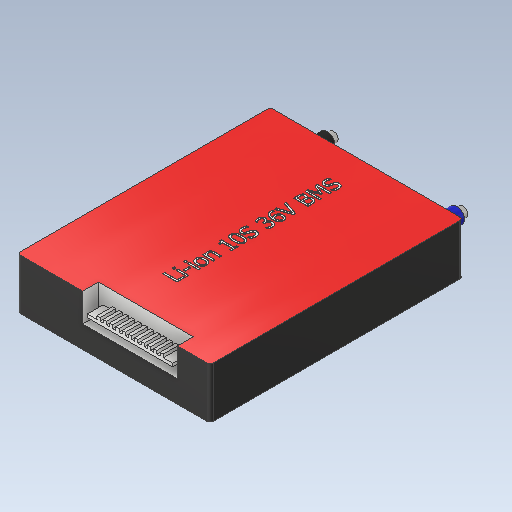
# Autodesk Inventor part: BMS
Saved by Autodesk Inventor 2020.1 (Build 241239000, 239)
## iProperties
Created: 2019-07-12
Part Number: BMS
Material: Generic
Document SubType Name: Modeling
Designer: Petar
Density: 1 g/cm^3
Appearance: Default
Author: Petar
Autodesk Inventor part; units mm, degrees
ref_plane "YZ Plane" through (0, 0, 0) normal (1, 0, 0) x (0, 1, 0)
ref_plane "XZ Plane" through (0, 0, 0) normal (0, 1, 0) x (-1, 0, 0)
ref_plane "XY Plane" through (0, 0, 0) normal (0, 0, 1) x (1, 0, 0)
sketch "Sketch1" plane through (0, 0, 0) normal (0, 1, 0) x (-1, 0, 0)
  line L0 (-30.5, 40) -> (30.5, 40)
  line L1 (30.5, 40) -> (30.5, -40)
  line L2 (30.5, -40) -> (-30.5, -40)
  line L3 (-30.5, -40) -> (-30.5, 40)
  line L4 (-30.5, 40) -> (30.5, -40) construction
  line L5 (30.5, 40) -> (-30.5, -40) construction
  point P0 (0, 0)
  dimension "d0" = 61
  dimension "d1" = 80
  constraints: 12 end point, 2 midpoint, 2 parallel, 1 horizontal, 1 perpendicular
  measures "d0" distance of L1.end L2.end
  measures "d1" distance of L0.end L1.end
extrude "Extrusion1" add sketch "Sketch1" along normal blind 16
sketch "Sketch2" plane through (0, 16, 0) normal (0, 1, 0) x (1, 0, 0)
  line L0 (-3.4837, -32.5737) -> (-3.4837, 39.7617) construction
  line L1 (-3.4837, 39.7617) -> (4.1906, 39.7617) construction
  line L2 (4.1906, 39.7617) -> (4.1906, -32.5737) construction
  line L3 (4.1906, -32.5737) -> (-3.4837, -32.5737) construction
  line L4 (-30.5, -40) -> (30.5, -40) construction
  line L5 (-9.8385, -40) -> (20.1615, -40)
  line L6 (20.1615, -40) -> (20.1615, -35)
  line L7 (20.1615, -35) -> (-9.8385, -35)
  line L8 (-9.8385, -35) -> (-9.8385, -40)
  line L9 (2.6034, -19.9781) -> (2.6034, -22.5855)
  line L10 (2.6034, -22.5855) -> (-1.8966, -22.5855)
  line L11 (-1.8966, -22.5855) -> (-1.8966, -21.9874)
  line L12 (-1.8966, -21.9874) -> (2.071, -21.9874)
  line L13 (2.071, -21.9874) -> (2.071, -19.9781)
  line L14 (2.071, -19.9781) -> (2.6034, -19.9781)
  line L15 (2.6034, -18.9716) -> (2.6034, -19.5405)
  line L16 (2.6034, -19.5405) -> (-0.7734, -19.5405)
  line L17 (-0.7734, -19.5405) -> (-0.7734, -18.9716)
  line L18 (-0.7734, -18.9716) -> (2.6034, -18.9716)
  line L19 (-1.335, -18.9315) -> (-1.335, -19.577)
  line L20 (-1.335, -19.577) -> (-1.9257, -19.577)
  line L21 (-1.9257, -19.577) -> (-1.9257, -18.9315)
  line L22 (-1.9257, -18.9315) -> (-1.335, -18.9315)
  line L23 (0.9077, -16.5721) -> (0.9077, -18.2751)
  line L24 (0.9077, -18.2751) -> (0.3607, -18.2751)
  line L25 (0.3607, -18.2751) -> (0.3607, -16.5721)
  line L26 (0.3607, -16.5721) -> (0.9077, -16.5721)
  line L27 (2.6034, -15.3104) -> (2.6034, -15.8793)
  line L28 (2.6034, -15.8793) -> (-0.7734, -15.8793)
  line L29 (-0.7734, -15.8793) -> (-0.7734, -15.3104)
  line L30 (-0.7734, -15.3104) -> (2.6034, -15.3104)
  line L31 (-1.335, -15.2703) -> (-1.335, -15.9157)
  line L32 (-1.335, -15.9157) -> (-1.9257, -15.9157)
  line L33 (-1.9257, -15.9157) -> (-1.9257, -15.2703)
  line L34 (-1.9257, -15.2703) -> (-1.335, -15.2703)
  spline S0 degree 2 poles (0.915, -11.7002) (1.7684, -11.7002) (2.6983, -12.5207) (2.6983, -13.2062) knots 0 0 0 1 2 2 2
  spline S1 degree 2 poles (2.6983, -13.2062) (2.6983, -13.9101) (1.7392, -14.716) (0.915, -14.716) knots 0 0 0 1 2 2 2
  spline S2 degree 2 poles (0.915, -14.716) (0.069, -14.716) (-0.8682, -13.8845) (-0.8682, -13.2062) knots 0 0 0 1 2 2 2
  spline S3 degree 2 poles (-0.8682, -13.2062) (-0.8682, -12.5207) (0.0654, -11.7002) (0.915, -11.7002) knots 0 0 0 1 2 2 2
  spline S4 degree 2 poles (0.915, -12.2873) (0.2586, -12.2873) (-0.3795, -12.765) (-0.3795, -13.2062) knots 0 0 0 1 2 2 2
  spline S5 degree 2 poles (-0.3795, -13.2062) (-0.3795, -13.6475) (0.2586, -14.1289) (0.915, -14.1289) knots 0 0 0 1 2 2 2
  spline S6 degree 2 poles (0.915, -14.1289) (1.5532, -14.1289) (2.2096, -13.6475) (2.2096, -13.2062) knots 0 0 0 1 2 2 2
  spline S7 degree 2 poles (2.2096, -13.2062) (2.2096, -12.7686) (1.5641, -12.2873) (0.915, -12.2873) knots 0 0 0 1 2 2 2
  line L35 (2.6034, -8.4656) -> (2.6034, -9.0344)
  line L36 (2.6034, -9.0344) -> (0.678, -9.0344)
  spline S8 degree 2 poles (0.678, -9.0344) (0.4446, -9.0344) (0.0435, -9.0782) (-0.0769, -9.1438) knots 0 0 0 1 2 2 2
  spline S9 degree 2 poles (-0.0769, -9.1438) (-0.2045, -9.2131) (-0.3285, -9.4611) (-0.3285, -9.6726) knots 0 0 0 1 2 2 2
  spline S10 degree 2 poles (-0.3285, -9.6726) (-0.3285, -9.8841) (-0.1024, -10.3327) (0.0799, -10.5478) knots 0 0 0 1 2 2 2
  line L37 (0.0799, -10.5478) -> (2.6034, -10.5478)
  line L38 (2.6034, -10.5478) -> (2.6034, -11.1167)
  line L39 (2.6034, -11.1167) -> (-0.7734, -11.1167)
  line L40 (-0.7734, -11.1167) -> (-0.7734, -10.5478)
  line L41 (-0.7734, -10.5478) -> (-0.3978, -10.5478)
  spline S11 degree 2 poles (-0.3978, -10.5478) (-0.6275, -10.2926) (-0.8682, -9.8003) (-0.8682, -9.5231) knots 0 0 0 1 2 2 2
  spline S12 degree 2 poles (-0.8682, -9.5231) (-0.8682, -9.0272) (-0.2118, -8.4656) (0.4118, -8.4656) knots 0 0 0 1 2 2 2
  line L42 (0.4118, -8.4656) -> (2.6034, -8.4656)
  line L43 (2.6034, -3.2691) -> (2.6034, -5.4644)
  line L44 (2.6034, -5.4644) -> (2.144, -5.4644)
  line L45 (2.144, -5.4644) -> (2.144, -4.6475)
  line L46 (2.144, -4.6475) -> (-0.8718, -4.6475)
  line L47 (-0.8718, -4.6475) -> (-0.8718, -5.4644)
  line L48 (-0.8718, -5.4644) -> (-1.2839, -5.4644)
  spline S13 degree 2 poles (-1.2839, -5.4644) (-1.2839, -5.0012) (-1.5465, -4.5636) (-1.9111, -4.5344) knots 0 0 0 1 2 2 2
  line L49 (-1.9111, -4.5344) -> (-1.9111, -4.0677)
  line L50 (-1.9111, -4.0677) -> (2.144, -4.0677)
  line L51 (2.144, -4.0677) -> (2.144, -3.2691)
  line L52 (2.144, -3.2691) -> (2.6034, -3.2691)
  spline S14 degree 2 poles (0.3534, 0.3594) (1.5641, 0.3594) (2.6983, -0.3444) (2.6983, -1.0774) knots 0 0 0 1 2 2 2
  spline S15 degree 2 poles (2.6983, -1.0774) (2.6983, -1.8213) (1.5423, -2.5178) (0.3571, -2.5178) knots 0 0 0 1 2 2 2
  spline S16 degree 2 poles (0.3571, -2.5178) (-0.8609, -2.5178) (-1.9877, -1.814) (-1.9877, -1.0774) knots 0 0 0 1 2 2 2
  spline S17 degree 2 poles (-1.9877, -1.0774) (-1.9877, -0.3371) (-0.8208, 0.3594) (0.3534, 0.3594) knots 0 0 0 1 2 2 2
  spline S18 degree 2 poles (1.7246, -0.4137) (1.5021, -0.3262) (0.8166, -0.2532) (0.3534, -0.2532) knots 0 0 0 1 2 2 2
  spline S19 degree 2 poles (0.3534, -0.2532) (-0.1097, -0.2532) (-0.7916, -0.3262) (-1.0214, -0.4173) knots 0 0 0 1 2 2 2
  spline S20 degree 2 poles (-1.0214, -0.4173) (-1.2511, -0.5085) (-1.4881, -0.8258) (-1.4881, -1.0774) knots 0 0 0 1 2 2 2
  spline S21 degree 2 poles (-1.4881, -1.0774) (-1.4881, -1.329) (-1.2511, -1.6536) (-1.0141, -1.7484) knots 0 0 0 1 2 2 2
  spline S22 degree 2 poles (-1.0141, -1.7484) (-0.7843, -1.8396) (-0.0842, -1.9052) (0.3571, -1.9052) knots 0 0 0 1 2 2 2
  spline S23 degree 2 poles (0.3571, -1.9052) (0.8312, -1.9052) (1.4657, -1.8468) (1.7137, -1.752) knots 0 0 0 1 2 2 2
  spline S24 degree 2 poles (1.7137, -1.752) (1.947, -1.6645) (2.1987, -1.34) (2.1987, -1.0774) knots 0 0 0 1 2 2 2
  spline S25 degree 2 poles (2.1987, -1.0774) (2.1987, -0.8294) (1.9616, -0.5049) (1.7246, -0.4137) knots 0 0 0 1 2 2 2
  spline S26 degree 2 poles (2.6837, 2.3177) (2.6837, 1.829) (2.4795, 1.1434) (2.3336, 0.8408) knots 0 0 0 1 2 2 2
  line L53 (2.3336, 0.8408) -> (1.5824, 0.8408)
  line L54 (1.5824, 0.8408) -> (1.5824, 0.8845)
  spline S27 degree 2 poles (1.5824, 0.8845) (1.8595, 1.1799) (2.1658, 1.9275) (2.1658, 2.2739) knots 0 0 0 1 2 2 2
  spline S28 degree 2 poles (2.1658, 2.2739) (2.1658, 2.7698) (1.7538, 3.2767) (1.4146, 3.2767) knots 0 0 0 1 2 2 2
  spline S29 degree 2 poles (1.4146, 3.2767) (1.1448, 3.2767) (0.8093, 3.0105) (0.7254, 2.7224) knots 0 0 0 1 2 2 2
  spline S30 degree 2 poles (0.7254, 2.7224) (0.6671, 2.5146) (0.5868, 2.1681) (0.5212, 1.9092) knots 0 0 0 1 2 2 2
  spline S31 degree 2 poles (0.5212, 1.9092) (0.4592, 1.6758) (0.2732, 1.3075) (0.1237, 1.1653) knots 0 0 0 1 2 2 2
  spline S32 degree 2 poles (0.1237, 1.1653) (-0.0258, 1.0267) (-0.4269, 0.8736) (-0.6895, 0.8736) knots 0 0 0 1 2 2 2
  spline S33 degree 2 poles (-0.6895, 0.8736) (-1.2365, 0.8736) (-1.9768, 1.7269) (-1.9768, 2.3869) knots 0 0 0 1 2 2 2
  spline S34 degree 2 poles (-1.9768, 2.3869) (-1.9768, 2.7662) (-1.8273, 3.4372) (-1.6851, 3.7253) knots 0 0 0 1 2 2 2
  line L55 (-1.6851, 3.7253) -> (-0.9703, 3.7253)
  line L56 (-0.9703, 3.7253) -> (-0.9703, 3.6815)
  spline S35 degree 2 poles (-0.9703, 3.6815) (-1.1672, 3.4664) (-1.459, 2.7954) (-1.459, 2.4271) knots 0 0 0 1 2 2 2
  spline S36 degree 2 poles (-1.459, 2.4271) (-1.459, 2.0113) (-1.0688, 1.4972) (-0.7515, 1.4972) knots 0 0 0 1 2 2 2
  spline S37 degree 2 poles (-0.7515, 1.4972) (-0.4671, 1.4972) (-0.1279, 1.7998) (-0.0513, 2.0843) knots 0 0 0 1 2 2 2
  spline S38 degree 2 poles (-0.0513, 2.0843) (-0.0003, 2.2739) (0.131, 2.8245) (0.1857, 3.0069) knots 0 0 0 1 2 2 2
  spline S39 degree 2 poles (0.1857, 3.0069) (0.3279, 3.47) (0.9004, 3.9003) (1.3198, 3.9003) knots 0 0 0 1 2 2 2
  spline S40 degree 2 poles (1.3198, 3.9003) (1.586, 3.9003) (2.0966, 3.6852) (2.2752, 3.4919) knots 0 0 0 1 2 2 2
  spline S41 degree 2 poles (2.2752, 3.4919) (2.4722, 3.2767) (2.6837, 2.7297) (2.6837, 2.3177) knots 0 0 0 1 2 2 2
  spline S42 degree 2 poles (-1.4699, 7.5288) (-1.4699, 7.3647) (-1.3897, 7.0401) (-1.3277, 6.8833) knots 0 0 0 1 2 2 2
  spline S43 degree 2 poles (-1.3277, 6.8833) (-1.2657, 6.7374) (-1.1344, 6.5223) (-1.0761, 6.4384) knots 0 0 0 1 2 2 2
  line L57 (-1.0761, 6.4384) -> (-1.0761, 6.4019)
  line L58 (-1.0761, 6.4019) -> (-1.7142, 6.4019)
  spline S44 degree 2 poles (-1.7142, 6.4019) (-1.82, 6.5989) (-1.9914, 7.2735) (-1.9914, 7.5762) knots 0 0 0 1 2 2 2
  spline S45 degree 2 poles (-1.9914, 7.5762) (-1.9914, 7.8825) (-1.8674, 8.3383) (-1.7361, 8.5243) knots 0 0 0 1 2 2 2
  spline S46 degree 2 poles (-1.7361, 8.5243) (-1.5939, 8.7212) (-1.1818, 8.9254) (-0.9047, 8.9254) knots 0 0 0 1 2 2 2
  spline S47 degree 2 poles (-0.9047, 8.9254) (-0.5327, 8.9254) (0.0289, 8.4368) (0.1018, 8.094) knots 0 0 0 1 2 2 2
  line L59 (0.1018, 8.094) -> (0.1456, 8.094)
  spline S48 degree 2 poles (0.1456, 8.094) (0.1748, 8.2362) (0.306, 8.5608) (0.4373, 8.6993) knots 0 0 0 1 2 2 2
  spline S49 degree 2 poles (0.4373, 8.6993) (0.5649, 8.8379) (0.9734, 9.013) (1.2688, 9.013) knots 0 0 0 1 2 2 2
  spline S50 degree 2 poles (1.2688, 9.013) (1.5714, 9.013) (2.0856, 8.8051) (2.2825, 8.6155) knots 0 0 0 1 2 2 2
  spline S51 degree 2 poles (2.2825, 8.6155) (2.4867, 8.4185) (2.6983, 7.8606) (2.6983, 7.5069) knots 0 0 0 1 2 2 2
  spline S52 degree 2 poles (2.6983, 7.5069) (2.6983, 7.1677) (2.5342, 6.504) (2.4211, 6.278) knots 0 0 0 1 2 2 2
  line L60 (2.4211, 6.278) -> (1.7829, 6.278)
  line L61 (1.7829, 6.278) -> (1.7829, 6.3217)
  spline S53 degree 2 poles (1.7829, 6.3217) (1.9215, 6.5113) (2.1768, 7.1532) (2.1768, 7.4704) knots 0 0 0 1 2 2 2
  spline S54 degree 2 poles (2.1768, 7.4704) (2.1768, 7.6564) (2.0601, 8.0284) (1.9252, 8.1523) knots 0 0 0 1 2 2 2
  spline S55 degree 2 poles (1.9252, 8.1523) (1.7902, 8.2727) (1.4693, 8.4003) (1.225, 8.4003) knots 0 0 0 1 2 2 2
  spline S56 degree 2 poles (1.225, 8.4003) (0.9807, 8.4003) (0.6634, 8.2581) (0.5722, 8.1305) knots 0 0 0 1 2 2 2
  spline S57 degree 2 poles (0.5722, 8.1305) (0.4811, 8.0028) (0.4118, 7.6564) (0.4118, 7.4522) knots 0 0 0 1 2 2 2
  line L62 (0.4118, 7.4522) -> (0.4118, 7.1969)
  line L63 (0.4118, 7.1969) -> (-0.0878, 7.1969)
  line L64 (-0.0878, 7.1969) -> (-0.0878, 7.3975)
  spline S58 degree 2 poles (-0.0878, 7.3975) (-0.0878, 7.8023) (-0.4744, 8.3128) (-0.8427, 8.3128) knots 0 0 0 1 2 2 2
  spline S59 degree 2 poles (-0.8427, 8.3128) (-1.0141, 8.3128) (-1.2584, 8.1815) (-1.3313, 8.0758) knots 0 0 0 1 2 2 2
  spline S60 degree 2 poles (-1.3313, 8.0758) (-1.4079, 7.9627) (-1.4699, 7.6856) (-1.4699, 7.5288) knots 0 0 0 1 2 2 2
  spline S61 degree 2 poles (1.1448, 12.5356) (1.4912, 12.5356) (2.0783, 12.3059) (2.2752, 12.1126) knots 0 0 0 1 2 2 2
  spline S62 degree 2 poles (2.2752, 12.1126) (2.4831, 11.9121) (2.6983, 11.4088) (2.6983, 11.1062) knots 0 0 0 1 2 2 2
  spline S63 degree 2 poles (2.6983, 11.1062) (2.6983, 10.8035) (2.494, 10.3039) (2.2898, 10.1143) knots 0 0 0 1 2 2 2
  spline S64 degree 2 poles (2.2898, 10.1143) (2.0455, 9.8809) (1.225, 9.6183) (0.6269, 9.6183) knots 0 0 0 1 2 2 2
  spline S65 degree 2 poles (0.6269, 9.6183) (0.0398, 9.6183) (-0.9047, 9.859) (-1.2547, 10.1106) knots 0 0 0 1 2 2 2
  spline S66 degree 2 poles (-1.2547, 10.1106) (-1.5975, 10.3549) (-1.9804, 11.128) (-1.9804, 11.6349) knots 0 0 0 1 2 2 2
  spline S67 degree 2 poles (-1.9804, 11.6349) (-1.9804, 11.7844) (-1.9513, 12.047) (-1.9184, 12.1455) knots 0 0 0 1 2 2 2
  line L65 (-1.9184, 12.1455) -> (-1.3386, 12.1455)
  line L66 (-1.3386, 12.1455) -> (-1.3386, 12.1199)
  spline S68 degree 2 poles (-1.3386, 12.1199) (-1.3824, 12.0361) (-1.459, 11.7297) (-1.459, 11.5547) knots 0 0 0 1 2 2 2
  spline S69 degree 2 poles (-1.459, 11.5547) (-1.459, 10.9931) (-0.7004, 10.3039) (0.0435, 10.2382) knots 0 0 0 1 2 2 2
  spline S70 degree 2 poles (0.0435, 10.2382) (-0.106, 10.4534) (-0.2701, 10.9056) (-0.2701, 11.1754) knots 0 0 0 1 2 2 2
  spline S71 degree 2 poles (-0.2701, 11.1754) (-0.2701, 11.438) (-0.1644, 11.8318) (-0.0039, 12.047) knots 0 0 0 1 2 2 2
  spline S72 degree 2 poles (-0.0039, 12.047) (0.182, 12.295) (0.7582, 12.5356) (1.1448, 12.5356) knots 0 0 0 1 2 2 2
  spline S73 degree 2 poles (1.1703, 11.923) (0.8931, 11.923) (0.5175, 11.7771) (0.3863, 11.6167) knots 0 0 0 1 2 2 2
  spline S74 degree 2 poles (0.3863, 11.6167) (0.2914, 11.4963) (0.2295, 11.1973) (0.2295, 11.0405) knots 0 0 0 1 2 2 2
  spline S75 degree 2 poles (0.2295, 11.0405) (0.2295, 10.829) (0.3571, 10.4315) (0.4774, 10.2382) knots 0 0 0 1 2 2 2
  spline S76 degree 2 poles (0.4774, 10.2382) (0.5431, 10.2346) (0.6671, 10.2273) (0.7619, 10.2273) knots 0 0 0 1 2 2 2
  spline S77 degree 2 poles (0.7619, 10.2273) (1.2286, 10.2273) (1.8012, 10.4096) (1.9507, 10.5482) knots 0 0 0 1 2 2 2
  spline S78 degree 2 poles (1.9507, 10.5482) (2.0929, 10.6758) (2.206, 10.953) (2.206, 11.1098) knots 0 0 0 1 2 2 2
  spline S79 degree 2 poles (2.206, 11.1098) (2.206, 11.4745) (1.6881, 11.923) (1.1703, 11.923) knots 0 0 0 1 2 2 2
  line L67 (-1.8966, 16.4595) -> (2.6034, 14.9096)
  line L68 (2.6034, 14.9096) -> (2.6034, 14.2642)
  line L69 (2.6034, 14.2642) -> (-1.8966, 12.7143)
  line L70 (-1.8966, 12.7143) -> (-1.8966, 13.3562)
  line L71 (-1.8966, 13.3562) -> (1.8413, 14.6033)
  line L72 (1.8413, 14.6033) -> (-1.8966, 15.8505)
  line L73 (-1.8966, 15.8505) -> (-1.8966, 16.4595)
  spline S80 degree 2 poles (1.2213, 21.8748) (1.5568, 21.8748) (2.071, 21.6195) (2.2388, 21.408) knots 0 0 0 1 2 2 2
  spline S81 degree 2 poles (2.2388, 21.408) (2.4357, 21.1527) (2.6034, 20.5729) (2.6034, 20.1134) knots 0 0 0 1 2 2 2
  line L74 (2.6034, 20.1134) -> (2.6034, 18.8225)
  line L75 (2.6034, 18.8225) -> (-1.8966, 18.8225)
  line L76 (-1.8966, 18.8225) -> (-1.8966, 20.015)
  spline S82 degree 2 poles (-1.8966, 20.015) (-1.8966, 20.4963) (-1.8346, 20.9777) (-1.7142, 21.1965) knots 0 0 0 1 2 2 2
  spline S83 degree 2 poles (-1.7142, 21.1965) (-1.5866, 21.4408) (-1.1672, 21.6633) (-0.8828, 21.6633) knots 0 0 0 1 2 2 2
  spline S84 degree 2 poles (-0.8828, 21.6633) (-0.5655, 21.6633) (-0.0623, 21.3278) (0.0799, 21.0324) knots 0 0 0 1 2 2 2
  line L77 (0.0799, 21.0324) -> (0.1018, 21.0324)
  spline S85 degree 2 poles (0.1018, 21.0324) (0.2112, 21.4335) (0.791, 21.8748) (1.2213, 21.8748) knots 0 0 0 1 2 2 2
  spline S86 degree 2 poles (1.2469, 21.2512) (0.9916, 21.2512) (0.6634, 21.1053) (0.5467, 20.8865) knots 0 0 0 1 2 2 2
  spline S87 degree 2 poles (0.5467, 20.8865) (0.4738, 20.7443) (0.43, 20.4088) (0.43, 20.0989) knots 0 0 0 1 2 2 2
  line L78 (0.43, 20.0989) -> (0.43, 19.4206)
  line L79 (0.43, 19.4206) -> (2.0929, 19.4206)
  line L80 (2.0929, 19.4206) -> (2.0929, 19.9056)
  spline S88 degree 2 poles (2.0929, 19.9056) (2.0929, 20.2994) (2.02, 20.7516) (1.9033, 20.9267) knots 0 0 0 1 2 2 2
  spline S89 degree 2 poles (1.9033, 20.9267) (1.7829, 21.0944) (1.4839, 21.2512) (1.2469, 21.2512) knots 0 0 0 1 2 2 2
  spline S90 degree 2 poles (-0.7989, 21.0397) (-0.9594, 21.0397) (-1.2, 20.9303) (-1.2693, 20.81) knots 0 0 0 1 2 2 2
  spline S91 degree 2 poles (-1.2693, 20.81) (-1.3496, 20.6641) (-1.386, 20.3104) (-1.386, 19.9931) knots 0 0 0 1 2 2 2
  line L81 (-1.386, 19.9931) -> (-1.386, 19.4206)
  line L82 (-1.386, 19.4206) -> (-0.0696, 19.4206)
  line L83 (-0.0696, 19.4206) -> (-0.0696, 20.0989)
  spline S92 degree 2 poles (-0.0696, 20.0989) (-0.0696, 20.3797) (-0.1279, 20.6459) (-0.2191, 20.7881) knots 0 0 0 1 2 2 2
  spline S93 degree 2 poles (-0.2191, 20.7881) (-0.3066, 20.9267) (-0.5874, 21.0397) (-0.7989, 21.0397) knots 0 0 0 1 2 2 2
  line L84 (2.6034, 26.3274) -> (2.6034, 25.7293)
  line L85 (2.6034, 25.7293) -> (-1.273, 25.7293)
  line L86 (-1.273, 25.7293) -> (1.3636, 24.5551)
  line L87 (1.3636, 24.5551) -> (1.3636, 24.1904)
  line L88 (1.3636, 24.1904) -> (-1.273, 23.0271)
  line L89 (-1.273, 23.0271) -> (2.6034, 23.0271)
  line L90 (2.6034, 23.0271) -> (2.6034, 22.4692)
  line L91 (2.6034, 22.4692) -> (-1.8966, 22.4692)
  line L92 (-1.8966, 22.4692) -> (-1.8966, 23.2861)
  line L93 (-1.8966, 23.2861) -> (0.6087, 24.4092)
  line L94 (0.6087, 24.4092) -> (-1.8966, 25.4959)
  line L95 (-1.8966, 25.4959) -> (-1.8966, 26.3274)
  line L96 (-1.8966, 26.3274) -> (2.6034, 26.3274)
  spline S94 degree 2 poles (2.6837, 28.4935) (2.6837, 28.0049) (2.4795, 27.3193) (2.3336, 27.0166) knots 0 0 0 1 2 2 2
  line L97 (2.3336, 27.0166) -> (1.5824, 27.0166)
  line L98 (1.5824, 27.0166) -> (1.5824, 27.0604)
  spline S95 degree 2 poles (1.5824, 27.0604) (1.8595, 27.3557) (2.1658, 28.1033) (2.1658, 28.4497) knots 0 0 0 1 2 2 2
  spline S96 degree 2 poles (2.1658, 28.4497) (2.1658, 28.9457) (1.7538, 29.4526) (1.4146, 29.4526) knots 0 0 0 1 2 2 2
  spline S97 degree 2 poles (1.4146, 29.4526) (1.1448, 29.4526) (0.8093, 29.1864) (0.7254, 28.8983) knots 0 0 0 1 2 2 2
  spline S98 degree 2 poles (0.7254, 28.8983) (0.6671, 28.6904) (0.5868, 28.344) (0.5212, 28.0851) knots 0 0 0 1 2 2 2
  spline S99 degree 2 poles (0.5212, 28.0851) (0.4592, 27.8517) (0.2732, 27.4834) (0.1237, 27.3412) knots 0 0 0 1 2 2 2
  spline S100 degree 2 poles (0.1237, 27.3412) (-0.0258, 27.2026) (-0.4269, 27.0494) (-0.6895, 27.0494) knots 0 0 0 1 2 2 2
  spline S101 degree 2 poles (-0.6895, 27.0494) (-1.2365, 27.0494) (-1.9768, 27.9027) (-1.9768, 28.5628) knots 0 0 0 1 2 2 2
  spline S102 degree 2 poles (-1.9768, 28.5628) (-1.9768, 28.942) (-1.8273, 29.613) (-1.6851, 29.9011) knots 0 0 0 1 2 2 2
  line L99 (-1.6851, 29.9011) -> (-0.9703, 29.9011)
  line L100 (-0.9703, 29.9011) -> (-0.9703, 29.8574)
  spline S103 degree 2 poles (-0.9703, 29.8574) (-1.1672, 29.6422) (-1.459, 28.9712) (-1.459, 28.6029) knots 0 0 0 1 2 2 2
  spline S104 degree 2 poles (-1.459, 28.6029) (-1.459, 28.1872) (-1.0688, 27.673) (-0.7515, 27.673) knots 0 0 0 1 2 2 2
  spline S105 degree 2 poles (-0.7515, 27.673) (-0.4671, 27.673) (-0.1279, 27.9757) (-0.0513, 28.2601) knots 0 0 0 1 2 2 2
  spline S106 degree 2 poles (-0.0513, 28.2601) (-0.0003, 28.4497) (0.131, 29.0004) (0.1857, 29.1827) knots 0 0 0 1 2 2 2
  spline S107 degree 2 poles (0.1857, 29.1827) (0.3279, 29.6459) (0.9004, 30.0762) (1.3198, 30.0762) knots 0 0 0 1 2 2 2
  spline S108 degree 2 poles (1.3198, 30.0762) (1.586, 30.0762) (2.0966, 29.861) (2.2752, 29.6677) knots 0 0 0 1 2 2 2
  spline S109 degree 2 poles (2.2752, 29.6677) (2.4722, 29.4526) (2.6837, 28.9056) (2.6837, 28.4935) knots 0 0 0 1 2 2 2
  point P0 (0, 0)
  dimension "d4" = 30
  dimension "d5" = 5
  constraints: 8 end point, 2 parallel, 1 horizontal, 1 perpendicular, 1 point on line, 2 other
  measures "d4" distance of L7.end L6.end
  measures "d5" distance of L6.end L5.end
extrude "Extrusion2" cut sketch "Sketch2" against normal blind 9 contours L8 L7 L6 L5
sketch "Sketch3" plane through (-9.8385, 16, 35) normal (0, 0, 1) x (1, 0, 0)
  line L0 (30, -9) -> (0, -9) construction
  line L1 (15, -9) -> (15, 0) construction
  line L2 (4.5, -4.5) -> (5.5, -4.5)
  line L3 (5.5, -4.5) -> (5.5, -5.5)
  line L4 (4.5, -5.5) -> (4.5, -4.5)
  line L5 (4.5, -6.5) -> (15, -6.5)
  line L6 (6.5, -5.5) -> (5.5, -5.5)
  line L7 (7.5, -5.5) -> (7.5, -4.5)
  line L8 (7.5, -4.5) -> (6.5, -4.5)
  line L9 (6.5, -4.5) -> (6.5, -5.5)
  line L10 (8.5, -5.5) -> (7.5, -5.5)
  line L11 (9.5, -5.5) -> (9.5, -4.5)
  line L12 (9.5, -4.5) -> (8.5, -4.5)
  line L13 (8.5, -4.5) -> (8.5, -5.5)
  line L14 (10.5, -5.5) -> (9.5, -5.5)
  line L15 (11.5, -5.5) -> (11.5, -4.5)
  line L16 (11.5, -4.5) -> (10.5, -4.5)
  line L17 (10.5, -4.5) -> (10.5, -5.5)
  line L18 (12.5, -5.5) -> (11.5, -5.5)
  line L19 (13.5, -5.5) -> (13.5, -4.5)
  line L20 (13.5, -4.5) -> (12.5, -4.5)
  line L21 (12.5, -4.5) -> (12.5, -5.5)
  line L22 (14.5, -5.5) -> (13.5, -5.5)
  line L23 (15, -6.5) -> (15, -4.5) construction
  line L24 (15, -4.5) -> (14.5, -4.5)
  line L25 (14.5, -4.5) -> (14.5, -5.5)
  line L26 (25.5, -4.5) -> (24.5, -4.5)
  line L27 (24.5, -4.5) -> (24.5, -5.5)
  line L28 (25.5, -6.5) -> (15, -6.5)
  line L29 (23.5, -5.5) -> (24.5, -5.5)
  line L30 (22.5, -5.5) -> (22.5, -4.5)
  line L31 (22.5, -4.5) -> (23.5, -4.5)
  line L32 (23.5, -4.5) -> (23.5, -5.5)
  line L33 (21.5, -5.5) -> (22.5, -5.5)
  line L34 (20.5, -5.5) -> (20.5, -4.5)
  line L35 (20.5, -4.5) -> (21.5, -4.5)
  line L36 (21.5, -4.5) -> (21.5, -5.5)
  line L37 (19.5, -5.5) -> (20.5, -5.5)
  line L38 (18.5, -5.5) -> (18.5, -4.5)
  line L39 (18.5, -4.5) -> (19.5, -4.5)
  line L40 (19.5, -4.5) -> (19.5, -5.5)
  line L41 (17.5, -5.5) -> (18.5, -5.5)
  line L42 (16.5, -5.5) -> (16.5, -4.5)
  line L43 (16.5, -4.5) -> (17.5, -4.5)
  line L44 (17.5, -4.5) -> (17.5, -5.5)
  line L45 (15.5, -5.5) -> (16.5, -5.5)
  line L46 (15.5, -4.5) -> (15.5, -5.5)
  line L47 (15.5, -4.5) -> (15, -4.5)
  line L48 (4.5, -5.5) -> (1.5, -5.5)
  line L49 (1.5, -5.5) -> (1.5, -6.5)
  line L50 (1.5, -6.5) -> (4.5, -6.5)
  line L51 (25.5, -6.5) -> (28.5, -6.5)
  line L52 (28.5, -6.5) -> (28.5, -5.5)
  line L53 (28.5, -5.5) -> (25.5, -5.5)
  line L54 (25.5, -5.5) -> (25.5, -4.5)
  point P0 (9.8385, -16)
  dimension "d12" = 1
  dimension "d13" = 1
  dimension "d14" = 0.5
  dimension "d15" = 2
  dimension "d16" = 1
  dimension "d17" = 2.5
  dimension "d20" = 3
  dimension "d21" = 3
  constraints: 108 end point, 22 symmetric about line, 15 collinear, 10 parallel, 6 perpendicular, 6 point on line, 5 horizontal, 2 vertical, 1 midpoint
  measures "d12" distance of L2.start L2.end
  measures "d13" distance of L6.start L3.end
  measures "d14" distance of L23.end L24.end
  measures "d15" distance of L5.start L2.start
  measures "d16" distance of L7.start L7.end
  measures "d17" distance between parallel lines of L0 L5
  measures "d20" distance of L5.start L49.end
  measures "d21" distance of L53.end L52.end
extrude "Extrusion3" add sketch "Sketch3" along normal blind 5
emboss "Emboss1" sketch "Sketch2" operation add depth 0.1 direction (0, -1, 0) contours L9 L10 L11 L12 L13 L14 | L15 L16 L17 L18 | L19 L20 L21 L22 | L23 L24 L25 L26 | L27 L28 L29 L30 | L31 L32 L33 L34 | S0 S1 S2 S3 | L35 L36 S8 S9 S10 L37 L38 L39 L40 L41 S11 S12 L42 | L43 L44 L45 L46 L47 L48 S13 L49 L50 L51 L52 | S14 S15 S16 S17 | S26 L53 L54 S27 S28 S29 S30 S31 S32 S33 S34 L55 L56 S35 S36 S37 S38 S39 S40 S41 | S42 S43 L57 L58 S44 S45 S46 S47 L59 S48 S49 S50 S51 S52 L60 L61 S53 S54 S55 S56 S57 L62 L63 L64 S58 S59 S60 | S61 S62 S63 S64 S65 S66 S67 L65 L66 S68 S69 S70 S71 S72 | L67 L68 L69 L70 L71 L72 L73 | S80 S81 L74 L75 L76 S82 S83 S84 L77 S85 | L84 L85 L86 L87 L88 L89 L90 L91 L92 L93 L94 L95 L96 | S94 L97 L98 S95 S96 S97 S98 S99 S100 S101 S102 L99 L100 S103 S104 S105 S106 S107 S108 S109
fillet "Fillet1" radius 1 4 edges at (30.5, 8, 40) (-30.5, 8, 40) (30.5, 8, -40) (-30.5, 8, -40)
sketch "Sketch4" plane through (29.5, 0, -40) normal (0, 0, -1) x (-1, 0, 0)
  circle A0 centre (9, 8) radius 2.5
  circle A1 centre (50, 8) radius 2.5
  line L0 (29.5, 0) -> (29.5, 16) construction
  line L1 (-1, 16) -> (-1, 0) construction
  line L2 (59, 0) -> (0, 0) construction
  circle A2 centre (9, 8) radius 1.53
  circle A3 centre (50, 8) radius 1.53
  line L3 (0, 16) -> (59, 16) construction
  dimension "d26" = 5
  dimension "d28" = 10
  dimension "d29" = 8
  dimension "d32" = 3.06
  constraints: 4 centre point, 2 end point, 2 symmetric about line, 1 coincident, 1 equal radius, 1 midpoint, 1 vertical, 1 other
  measures "d26" diameter of A0
  measures "d28" distance from line of L1 A0.centre
  measures "d29" distance from line of L2 A0.centre
  measures "d32" diameter of A2
extrude "Extrusion4" add sketch "Sketch4" along normal blind 8 contours A0 | A1 | A2 | A3
extrude "Extrusion5" add sketch "Sketch4" along normal blind 10 contours A2 | A3
body "Solid1"
